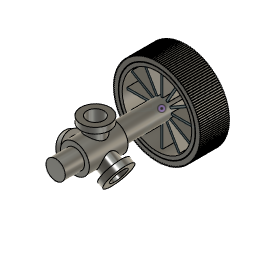
Inner Rotor Generator + Hub (Autodesk Fusion 360 design; units mm, degrees)
Autodesk Fusion 360 part; units mm, degrees
(part 1 of 2)
sketch "Sketch1" plane through (0, 0, 0) normal (0, 1, 0) x (1, 0, 0) in component "Inner Rotor Generator"
  circle A0 centre (0, 0) radius 4500
  circle A1 centre (0, 0) radius 4000
  circle A2 centre (0, 0) radius 1000
  circle A3 centre (0, 0) radius 3950
  circle A4 centre (0, 0) radius 3600
  line L0 (-100, -900) -> (100, -900)
  line L1 (100, -900) -> (100, -3700)
  line L2 (100, -3700) -> (-100, -3700)
  line L3 (-100, -3700) -> (-100, -900)
  line L4 (20.1805, -4430.0009) -> (-19.8217, -4429.9984)
  line L5 (-19.8217, -4429.9984) -> (-19.8172, -4499.9564)
  line L6 (20.176, -4499.9548) -> (20.1805, -4430.0009)
  line L7 (-19.8172, -4499.9564) -> (20.176, -4499.9548)
  line L8 (165.7048, -4426.9426) -> (168.6388, -4496.839)
  line L9 (168.6388, -4496.839) -> (208.5969, -4495.1627)
  line L10 (208.5969, -4495.1627) -> (205.6719, -4425.27)
  line L11 (205.6719, -4425.27) -> (165.7048, -4426.9426)
  line L12 (350.9405, -4416.1204) -> (356.7989, -4485.8326)
  line L13 (356.7989, -4485.8326) -> (396.6518, -4482.4845)
  line L14 (396.6518, -4482.4845) -> (390.8026, -4412.7756)
  line L15 (390.8026, -4412.7756) -> (350.9405, -4416.1204)
  line L16 (535.5606, -4397.5508) -> (544.3331, -4466.9566)
  line L17 (544.3331, -4466.9566) -> (584.0108, -4461.9426)
  line L18 (584.0108, -4461.9426) -> (575.2477, -4392.5398)
  line L19 (575.2477, -4392.5398) -> (535.5606, -4397.5508)
  line L20 (719.2411, -4371.2665) -> (730.9124, -4440.244)
  line L21 (730.9124, -4440.244) -> (770.3453, -4433.5728)
  line L22 (770.3453, -4433.5728) -> (758.6836, -4364.5979)
  line L23 (758.6836, -4364.5979) -> (719.2411, -4371.2665)
  line L24 (901.6599, -4337.3135) -> (916.2094, -4405.7417)
  line L25 (916.2094, -4405.7417) -> (955.3283, -4397.4251)
  line L26 (955.3283, -4397.4251) -> (940.7885, -4328.999)
  line L27 (940.7885, -4328.999) -> (901.6599, -4337.3135)
  line L28 (1082.4968, -4295.7513) -> (1099.899, -4363.5103)
  line L29 (1099.899, -4363.5103) -> (1138.6354, -4353.5628)
  line L30 (1138.6354, -4353.5628) -> (1121.2429, -4285.8056)
  line L31 (1121.2429, -4285.8056) -> (1082.4968, -4295.7513)
  line L32 (1261.4347, -4246.6529) -> (1281.6591, -4313.6238)
  line L33 (1281.6591, -4313.6238) -> (1319.9449, -4302.0629)
  line L34 (1319.9449, -4302.0629) -> (1299.7303, -4235.0935)
  line L35 (1299.7303, -4235.0935) -> (1261.4347, -4246.6529)
  line L36 (1438.1596, -4190.1045) -> (1461.1707, -4256.1697)
  line L37 (1461.1707, -4256.1697) -> (1498.9388, -4243.0157)
  line L38 (1498.9388, -4243.0157) -> (1475.9375, -4176.9515)
  line L39 (1475.9375, -4176.9515) -> (1438.1596, -4190.1045)
  line L40 (1612.3614, -4126.2052) -> (1638.1189, -4191.2488)
  line L41 (1638.1189, -4191.2488) -> (1675.303, -4176.5248)
  line L42 (1675.303, -4176.5248) -> (1649.5554, -4111.4818)
  line L43 (1649.5554, -4111.4818) -> (1612.3614, -4126.2052)
  line L44 (1783.7346, -4055.0671) -> (1812.1932, -4118.9751)
  line L45 (1812.1932, -4118.9751) -> (1848.7282, -4102.7069)
  line L46 (1848.7282, -4102.7069) -> (1820.2795, -4038.7991)
  line L47 (1820.2795, -4038.7991) -> (1783.7346, -4055.0671)
  line L48 (1951.9786, -3976.8151) -> (1983.0884, -4039.4753)
  line L49 (1983.0884, -4039.4753) -> (2018.9101, -4021.6914)
  line L50 (2018.9101, -4021.6914) -> (1987.8101, -3959.031)
  line L51 (1987.8101, -3959.031) -> (1951.9786, -3976.8151)
  line L52 (2116.7981, -3891.5864) -> (2150.5046, -3952.8888)
  line L53 (2150.5046, -3952.8888) -> (2185.5501, -3933.6205)
  line L54 (2185.5501, -3933.6205) -> (2151.8535, -3872.3174)
  line L55 (2151.8535, -3872.3174) -> (2116.7981, -3891.5864)
  line L56 (2277.904, -3799.5305) -> (2314.148, -3859.3677)
  line L57 (2314.148, -3859.3677) -> (2348.356, -3838.6488)
  line L58 (2348.356, -3838.6488) -> (2312.1218, -3778.8104)
  line L59 (2312.1218, -3778.8104) -> (2277.904, -3799.5305)
  line L60 (2435.0137, -3700.8089) -> (2473.7317, -3759.0759)
  line L61 (2473.7317, -3759.0759) -> (2507.042, -3736.9427)
  line L62 (2507.042, -3736.9427) -> (2468.3338, -3678.6742)
  line L63 (2468.3338, -3678.6742) -> (2435.0137, -3700.8089)
  line L64 (2587.8516, -3595.5949) -> (2628.9755, -3652.1894)
  line L65 (2628.9755, -3652.1894) -> (2661.3298, -3628.6807)
  line L66 (2661.3298, -3628.6807) -> (2620.2156, -3572.0843)
  line L67 (2620.2156, -3572.0843) -> (2587.8516, -3595.5949)
  line L68 (2736.1495, -3484.073) -> (2779.6073, -3538.8958)
  line L69 (2779.6073, -3538.8958) -> (2810.9487, -3514.0528)
  line L70 (2810.9487, -3514.0528) -> (2767.5005, -3459.2277)
  line L71 (2767.5005, -3459.2277) -> (2736.1495, -3484.073)
  line L72 (2879.6473, -3366.4388) -> (2925.3627, -3419.3937)
  line L73 (2925.3627, -3419.3937) -> (2955.6363, -3393.2601)
  line L74 (2955.6363, -3393.2601) -> (2909.9304, -3340.3025)
  line L75 (2909.9304, -3340.3025) -> (2879.6473, -3366.4388)
  line L76 (3018.0932, -3242.8987) -> (3065.986, -3293.8928)
  line L77 (3065.986, -3293.8928) -> (3095.1387, -3266.5144)
  line L78 (3095.1387, -3266.5144) -> (3047.2552, -3215.5172)
  line L79 (3047.2552, -3215.5172) -> (3018.0932, -3242.8987)
  line L80 (3151.2443, -3113.6695) -> (3201.2305, -3162.6133)
  line L81 (3201.2305, -3162.6133) -> (3229.2112, -3134.0382)
  line L82 (3229.2112, -3134.0382) -> (3179.2342, -3085.0909)
  line L83 (3179.2342, -3085.0909) -> (3151.2443, -3113.6695)
  line L84 (3278.8671, -2978.9779) -> (3330.859, -3025.7856)
  line L85 (3330.859, -3025.7856) -> (3357.6185, -2996.0637)
  line L86 (3357.6185, -2996.0637) -> (3305.6356, -2949.2522)
  line L87 (3305.6356, -2949.2522) -> (3278.8671, -2978.9779)
  line L88 (3400.7376, -2839.0601) -> (3454.644, -2883.6496)
  line L89 (3454.644, -2883.6496) -> (3480.1354, -2852.8332)
  line L90 (3480.1354, -2852.8332) -> (3426.2379, -2808.2395)
  line L91 (3426.2379, -2808.2395) -> (3400.7376, -2839.0601)
  line L92 (3516.6421, -2694.1617) -> (3572.3684, -2736.4546)
  line L93 (3572.3684, -2736.4546) -> (3596.547, -2704.5979)
  line L94 (3596.547, -2704.5979) -> (3540.8294, -2662.3003)
  line L95 (3540.8294, -2662.3003) -> (3516.6421, -2694.1617)
  line L96 (3626.3772, -2544.5368) -> (3683.8257, -2584.459)
  line L97 (3683.8257, -2584.459) -> (3706.649, -2551.6177)
  line L98 (3706.649, -2551.6177) -> (3649.209, -2511.6905)
  line L99 (3649.209, -2511.6905) -> (3626.3772, -2544.5368)
  line L100 (3729.7503, -2390.4479) -> (3788.8202, -2427.9294)
  line L101 (3788.8202, -2427.9294) -> (3810.2483, -2394.1612)
  line L102 (3810.2483, -2394.1612) -> (3751.1867, -2356.6743)
  line L103 (3751.1867, -2356.6743) -> (3729.7503, -2390.4479)
  line L104 (3826.5803, -2232.1653) -> (3887.1679, -2267.1404)
  line L105 (3887.1679, -2267.1404) -> (3907.1632, -2232.5044)
  line L106 (3907.1632, -2232.5044) -> (3846.5836, -2197.5237)
  line L107 (3846.5836, -2197.5237) -> (3826.5803, -2232.1653)
  line L108 (3916.6971, -2069.9668) -> (3978.6962, -2102.374)
  line L109 (3978.6962, -2102.374) -> (3997.2235, -2066.9311)
  line L110 (3997.2235, -2066.9311) -> (3935.2322, -2034.5179)
  line L111 (3935.2322, -2034.5179) -> (3916.6971, -2069.9668)
  line L112 (3999.9427, -1904.1368) -> (4063.2445, -1933.9194)
  line L113 (4063.2445, -1933.9194) -> (4080.2713, -1897.7317)
  line L114 (4080.2713, -1897.7317) -> (4016.9771, -1867.9428)
  line L115 (4016.9771, -1867.9428) -> (3999.9427, -1904.1368)
  line L116 (4076.1711, -1734.9663) -> (4140.6645, -1762.072)
  line L117 (4140.6645, -1762.072) -> (4156.161, -1725.2031)
  line L118 (4156.161, -1725.2031) -> (4091.6749, -1698.0908)
  line L119 (4091.6749, -1698.0908) -> (4076.1711, -1734.9663)
  line L120 (4145.2484, -1562.7521) -> (4210.8203, -1587.1333)
  line L121 (4210.8203, -1587.1333) -> (4224.7594, -1549.6478)
  line L122 (4224.7594, -1549.6478) -> (4159.1944, -1525.2597)
  line L123 (4159.1944, -1525.2597) -> (4145.2484, -1562.7521)
  line L124 (4207.0536, -1387.7964) -> (4273.589, -1409.4103)
  line L125 (4273.589, -1409.4103) -> (4285.946, -1371.3739)
  line L126 (4285.946, -1371.3739) -> (4219.4174, -1349.7528)
  line L127 (4219.4174, -1349.7528) -> (4207.0536, -1387.7964)
  line L128 (4261.4782, -1210.4059) -> (4328.8603, -1229.2146)
  line L129 (4328.8603, -1229.2146) -> (4339.6137, -1190.6942)
  line L130 (4339.6137, -1190.6942) -> (4272.238, -1171.878)
  line L131 (4272.238, -1171.878) -> (4261.4782, -1210.4059)
  line L132 (4308.4267, -1030.892) -> (4376.5373, -1046.8626)
  line L133 (4376.5373, -1046.8626) -> (4385.6682, -1007.9256)
  line L134 (4385.6682, -1007.9256) -> (4317.5637, -991.9473)
  line L135 (4317.5637, -991.9473) -> (4308.4267, -1030.892)
  line L136 (4347.8167, -849.5695) -> (4416.5364, -862.6739)
  line L137 (4416.5364, -862.6739) -> (4424.0288, -823.3888)
  line L138 (4424.0288, -823.3888) -> (4355.3149, -810.2764)
  line L139 (4355.3149, -810.2764) -> (4347.8167, -849.5695)
  line L140 (4379.5792, -666.7567) -> (4448.7874, -676.9719)
  line L141 (4448.7874, -676.9719) -> (4454.6281, -637.4074)
  line L142 (4454.6281, -637.4074) -> (4385.4254, -627.184)
  line L143 (4385.4254, -627.184) -> (4379.5792, -666.7567)
  line L144 (4403.6585, -482.7741) -> (4473.2337, -490.0822)
  line L145 (4473.2337, -490.0822) -> (4477.4125, -450.3078)
  line L146 (4477.4125, -450.3078) -> (4407.8423, -442.9913)
  line L147 (4407.8423, -442.9913) -> (4403.6585, -482.7741)
  line L148 (4420.0122, -297.9445) -> (4489.8324, -302.3327)
  line L149 (4489.8324, -302.3327) -> (4492.342, -262.4183)
  line L150 (4492.342, -262.4183) -> (4422.5265, -258.0214)
  line L151 (4422.5265, -258.0214) -> (4420.0122, -297.9445)
  line L152 (4428.6117, -112.5923) -> (4498.5544, -114.0528)
  line L153 (4498.5544, -114.0528) -> (4499.3904, -74.0683)
  line L154 (4499.3904, -74.0683) -> (4429.452, -72.5989)
  line L155 (4429.452, -72.5989) -> (4428.6117, -112.5923)
  line L156 (4429.4419, 72.9575) -> (4499.3845, 74.4271)
  line L157 (4499.3845, 74.4271) -> (4498.5453, 114.4116)
  line L158 (4498.5453, 114.4116) -> (4428.6067, 112.951)
  line L159 (4428.6067, 112.951) -> (4429.4419, 72.9575)
  line L160 (4422.5014, 258.3793) -> (4492.3211, 262.7765)
  line L161 (4492.3211, 262.7765) -> (4489.8083, 302.6907)
  line L162 (4489.8083, 302.6907) -> (4419.9922, 298.3027)
  line L163 (4419.9922, 298.3027) -> (4422.5014, 258.3793)
  line L164 (4407.8023, 443.3478) -> (4477.3766, 450.6649)
  line L165 (4477.3766, 450.6649) -> (4473.1946, 490.4389)
  line L166 (4473.1946, 490.4389) -> (4403.6235, 483.1311)
  line L167 (4403.6235, 483.1311) -> (4407.8023, 443.3478)
  line L168 (4385.3705, 627.5385) -> (4454.5773, 637.7626)
  line L169 (4454.5773, 637.7626) -> (4448.7334, 677.3266)
  line L170 (4448.7334, 677.3266) -> (4379.5293, 667.1119)
  line L171 (4379.5293, 667.1119) -> (4385.3705, 627.5385)
  line L172 (4355.2452, 810.6283) -> (4423.9631, 823.7416)
  line L173 (4423.9631, 823.7416) -> (4416.4676, 863.0261)
  line L174 (4416.4676, 863.0261) -> (4347.752, 849.9224)
  line L175 (4347.752, 849.9224) -> (4355.2452, 810.6283)
  line L176 (4317.4793, 992.296) -> (4385.5879, 1008.2753)
  line L177 (4385.5879, 1008.2753) -> (4376.4538, 1047.2115)
  line L178 (4376.4538, 1047.2115) -> (4308.3472, 1031.2418)
  line L179 (4308.3472, 1031.2418) -> (4317.4793, 992.296)
  line L180 (4272.1391, 1172.2228) -> (4339.5188, 1191.0403)
  line L181 (4339.5188, 1191.0403) -> (4328.7623, 1229.5598)
  line L182 (4328.7623, 1229.5598) -> (4261.3841, 1210.7521)
  line L183 (4261.3841, 1210.7521) -> (4272.1391, 1172.2228)
  line L184 (4219.3041, 1350.0932) -> (4285.8367, 1371.7157)
  line L185 (4285.8367, 1371.7157) -> (4273.4766, 1409.751)
  line L186 (4273.4766, 1409.751) -> (4206.9451, 1388.1383)
  line L187 (4206.9451, 1388.1383) -> (4219.3041, 1350.0932)
  line L188 (4159.067, 1525.5951) -> (4224.6358, 1549.9847)
  line L189 (4224.6358, 1549.9847) -> (4210.6938, 1587.4691)
  line L190 (4210.6938, 1587.4691) -> (4145.1257, 1563.0893)
  line L191 (4145.1257, 1563.0893) -> (4159.067, 1525.5951)
  line L192 (4091.5335, 1698.4205) -> (4156.0234, 1725.5345)
  line L193 (4156.0234, 1725.5345) -> (4140.524, 1762.4022)
  line L194 (4140.524, 1762.4022) -> (4076.0344, 1735.298)
  line L195 (4076.0344, 1735.298) -> (4091.5335, 1698.4205)
  line L196 (4016.8221, 1868.2664) -> (4080.12, 1898.0571)
  line L197 (4080.12, 1898.0571) -> (4063.0903, 1934.2434)
  line L198 (4063.0903, 1934.2434) -> (3999.7923, 1904.4625)
  line L199 (3999.7923, 1904.4625) -> (4016.8221, 1868.2664)
  line L200 (3935.0638, 2034.8346) -> (3997.0587, 2067.2499)
  line L201 (3997.0587, 2067.2499) -> (3978.5285, 2102.6913)
  line L202 (3978.5285, 2102.6913) -> (3916.5331, 2070.2859)
  line L203 (3916.5331, 2070.2859) -> (3935.0638, 2034.8346)
  line L204 (3846.402, 2197.8331) -> (3906.9851, 2232.816)
  line L205 (3906.9851, 2232.816) -> (3886.9871, 2267.4503)
  line L206 (3886.9871, 2267.4503) -> (3826.4031, 2232.4773)
  line L207 (3826.4031, 2232.4773) -> (3846.402, 2197.8331)
  line L208 (3750.9924, 2356.9758) -> (3810.0574, 2394.465)
  line L209 (3810.0574, 2394.465) -> (3788.6266, 2428.2315)
  line L210 (3788.6266, 2428.2315) -> (3729.5603, 2390.7521)
  line L211 (3729.5603, 2390.7521) -> (3750.9924, 2356.9758)
  line L212 (3649.0022, 2511.9836) -> (3706.4456, 2551.9133)
  line L213 (3706.4456, 2551.9133) -> (3683.6196, 2584.7528)
  line L214 (3683.6196, 2584.7528) -> (3626.1745, 2544.8328)
  line L215 (3626.1745, 2544.8328) -> (3649.0022, 2511.9836)
  line L216 (3540.6104, 2662.5845) -> (3596.3313, 2704.8846)
  line L217 (3596.3313, 2704.8846) -> (3572.1502, 2736.7395)
  line L218 (3572.1502, 2736.7395) -> (3516.4272, 2694.449)
  line L219 (3516.4272, 2694.449) -> (3540.6104, 2662.5845)
  line L220 (3426.0073, 2808.5144) -> (3479.9079, 2853.1107)
  line L221 (3479.9079, 2853.1107) -> (3454.4141, 2883.925)
  line L222 (3454.4141, 2883.925) -> (3400.5109, 2839.3382)
  line L223 (3400.5109, 2839.3382) -> (3426.0073, 2808.5144)
  line L224 (3305.3937, 2949.5171) -> (3357.3796, 2996.3315)
  line L225 (3357.3796, 2996.3315) -> (3330.6177, 3026.0512)
  line L226 (3330.6177, 3026.0512) -> (3278.6289, 2979.2462)
  line L227 (3278.6289, 2979.2462) -> (3305.3937, 2949.5171)
  line L228 (3178.9813, 3085.3454) -> (3228.9612, 3134.2957)
  line L229 (3228.9612, 3134.2957) -> (3200.9783, 3162.8686)
  line L230 (3200.9783, 3162.8686) -> (3150.9951, 3113.9276)
  line L231 (3150.9951, 3113.9276) -> (3178.9813, 3085.3454)
  line L232 (3046.992, 3215.7609) -> (3094.8782, 3266.7612)
  line L233 (3094.8782, 3266.7612) -> (3065.7233, 3294.1373)
  line L234 (3065.7233, 3294.1373) -> (3017.8334, 3243.1462)
  line L235 (3017.8334, 3243.1462) -> (3046.992, 3215.7609)
  line L236 (2909.6572, 3340.535) -> (2955.3657, 3393.4958)
  line L237 (2955.3657, 3393.4958) -> (2925.09, 3419.6269)
  line L238 (2925.09, 3419.6269) -> (2879.3774, 3366.6751)
  line L239 (2879.3774, 3366.6751) -> (2909.6572, 3340.535)
  line L240 (2767.2178, 3459.4485) -> (2810.6685, 3514.277)
  line L241 (2810.6685, 3514.277) -> (2779.3251, 3539.1174)
  line L242 (2779.3251, 3539.1174) -> (2735.8699, 3484.2978)
  line L243 (2735.8699, 3484.2978) -> (2767.2178, 3459.4485)
  line L244 (2619.9238, 3572.2931) -> (2661.0404, 3628.8929)
  line L245 (2661.0404, 3628.8929) -> (2628.6843, 3652.3991)
  line L246 (2628.6843, 3652.3991) -> (2587.5629, 3595.8078)
  line L247 (2587.5629, 3595.8078) -> (2619.9238, 3572.2931)
  line L248 (2468.0336, 3678.8706) -> (2506.744, 3737.1426)
  line L249 (2506.744, 3737.1426) -> (2473.4319, 3759.2732)
  line L250 (2473.4319, 3759.2732) -> (2434.7163, 3701.0096)
  line L251 (2434.7163, 3701.0096) -> (2468.0336, 3678.8706)
  line L252 (2311.8136, 3778.9941) -> (2348.0499, 3838.836)
  line L253 (2348.0499, 3838.836) -> (2313.8403, 3859.5522)
  line L254 (2313.8403, 3859.5522) -> (2277.5985, 3799.7185)
  line L255 (2277.5985, 3799.7185) -> (2311.8136, 3778.9941)
  line L256 (2151.5379, 3872.488) -> (2185.2365, 3933.7948)
  line L257 (2185.2365, 3933.7948) -> (2150.1894, 3953.0603)
  line L258 (2150.1894, 3953.0603) -> (2116.4849, 3891.7614)
  line L259 (2116.4849, 3891.7614) -> (2151.5379, 3872.488)
  line L260 (1987.4877, 3959.1882) -> (2018.5894, 4021.8524)
  line L261 (2018.5894, 4021.8524) -> (1982.7663, 4039.6334)
  line L262 (1982.7663, 4039.6334) -> (1951.6584, 3976.9769)
  line L263 (1951.6584, 3976.9769) -> (1987.4877, 3959.1882)
  line L264 (1819.9507, 4038.9427) -> (1848.4011, 4102.8543)
  line L265 (1848.4011, 4102.8543) -> (1811.8648, 4119.1196)
  line L266 (1811.8648, 4119.1196) -> (1783.4079, 4055.2154)
  line L267 (1783.4079, 4055.2154) -> (1819.9507, 4038.9427)
  line L268 (1649.2209, 4111.6115) -> (1674.97, 4176.6584)
  line L269 (1674.97, 4176.6584) -> (1637.7846, 4191.3794)
  line L270 (1637.7846, 4191.3794) -> (1612.0288, 4126.3396)
  line L271 (1612.0288, 4126.3396) -> (1649.2209, 4111.6115)
  line L272 (1475.5979, 4177.0671) -> (1498.6005, 4243.1352)
  line L273 (1498.6005, 4243.1352) -> (1460.8313, 4256.2862)
  line L274 (1460.8313, 4256.2862) -> (1437.8216, 4190.2249)
  line L275 (1437.8216, 4190.2249) -> (1475.5979, 4177.0671)
  line L276 (1299.3861, 4235.1947) -> (1319.6019, 4302.1682)
  line L277 (1319.6019, 4302.1682) -> (1281.3151, 4313.726)
  line L278 (1281.3151, 4313.726) -> (1261.092, 4246.7591)
  line L279 (1261.092, 4246.7591) -> (1299.3861, 4235.1947)
  line L280 (1120.8948, 4285.8924) -> (1138.2882, 4353.6536)
  line L281 (1138.2882, 4353.6536) -> (1099.5511, 4363.598)
  line L282 (1099.5511, 4363.598) -> (1082.15, 4295.843)
  line L283 (1082.15, 4295.843) -> (1120.8948, 4285.8924)
  line L284 (940.437, 4329.0711) -> (954.9777, 4397.5013)
  line L285 (954.9777, 4397.5013) -> (915.8581, 4405.8148)
  line L286 (915.8581, 4405.8148) -> (901.3095, 4337.3905)
  line L287 (901.3095, 4337.3905) -> (940.437, 4329.0711)
  line L288 (758.3294, 4364.6552) -> (769.9918, 4433.6343)
  line L289 (769.9918, 4433.6343) -> (730.5583, 4440.3023)
  line L290 (730.5583, 4440.3023) -> (718.8878, 4371.3288)
  line L291 (718.8878, 4371.3288) -> (758.3294, 4364.6552)
  line L292 (574.8914, 4392.5822) -> (583.655, 4461.9891)
  line L293 (583.655, 4461.9891) -> (543.9769, 4467)
  line L294 (543.9769, 4467) -> (535.205, 4397.5983)
  line L295 (535.205, 4397.5983) -> (574.8914, 4392.5822)
  line L296 (390.4449, 4412.8031) -> (396.2943, 4482.5161)
  line L297 (396.2943, 4482.5161) -> (356.4412, 4485.8611)
  line L298 (356.4412, 4485.8611) -> (350.5832, 4416.1529)
  line L299 (350.5832, 4416.1529) -> (390.4449, 4412.8031)
  line L300 (205.3134, 4425.2825) -> (208.2384, 4495.1793)
  line L301 (208.2384, 4495.1793) -> (168.2802, 4496.8524)
  line L302 (168.2802, 4496.8524) -> (165.3464, 4426.9601)
  line L303 (165.3464, 4426.9601) -> (205.3134, 4425.2825)
  line L304 (19.8217, 4429.9984) -> (19.8172, 4499.9564)
  line L305 (19.8172, 4499.9564) -> (-20.176, 4499.9548)
  line L306 (-20.176, 4499.9548) -> (-20.1805, 4430.0009)
  line L307 (-20.1805, 4430.0009) -> (19.8217, 4429.9984)
  line L308 (-165.7048, 4426.9426) -> (-168.6388, 4496.839)
  line L309 (-168.6388, 4496.839) -> (-208.5969, 4495.1627)
  line L310 (-208.5969, 4495.1627) -> (-205.6719, 4425.27)
  line L311 (-205.6719, 4425.27) -> (-165.7048, 4426.9426)
  line L312 (-350.9405, 4416.1204) -> (-356.7989, 4485.8326)
  line L313 (-356.7989, 4485.8326) -> (-396.6518, 4482.4845)
  line L314 (-396.6518, 4482.4845) -> (-390.8026, 4412.7756)
  line L315 (-390.8026, 4412.7756) -> (-350.9405, 4416.1204)
  line L316 (-535.5606, 4397.5508) -> (-544.3331, 4466.9566)
  line L317 (-544.3331, 4466.9566) -> (-584.0108, 4461.9426)
  line L318 (-584.0108, 4461.9426) -> (-575.2477, 4392.5398)
  line L319 (-575.2477, 4392.5398) -> (-535.5606, 4397.5508)
  line L320 (-719.2411, 4371.2665) -> (-730.9124, 4440.244)
  line L321 (-730.9124, 4440.244) -> (-770.3453, 4433.5728)
  line L322 (-770.3453, 4433.5728) -> (-758.6836, 4364.5979)
  line L323 (-758.6836, 4364.5979) -> (-719.2411, 4371.2665)
  line L324 (-901.6599, 4337.3135) -> (-916.2094, 4405.7417)
  line L325 (-916.2094, 4405.7417) -> (-955.3283, 4397.4251)
  line L326 (-955.3283, 4397.4251) -> (-940.7885, 4328.999)
  line L327 (-940.7885, 4328.999) -> (-901.6599, 4337.3135)
  line L328 (-1082.4968, 4295.7513) -> (-1099.899, 4363.5103)
  line L329 (-1099.899, 4363.5103) -> (-1138.6354, 4353.5628)
  line L330 (-1138.6354, 4353.5628) -> (-1121.2429, 4285.8056)
  line L331 (-1121.2429, 4285.8056) -> (-1082.4968, 4295.7513)
  line L332 (-1261.4347, 4246.6529) -> (-1281.6591, 4313.6238)
  line L333 (-1281.6591, 4313.6238) -> (-1319.9449, 4302.0629)
  line L334 (-1319.9449, 4302.0629) -> (-1299.7303, 4235.0935)
  line L335 (-1299.7303, 4235.0935) -> (-1261.4347, 4246.6529)
  line L336 (-1438.1596, 4190.1045) -> (-1461.1707, 4256.1697)
  line L337 (-1461.1707, 4256.1697) -> (-1498.9388, 4243.0157)
  line L338 (-1498.9388, 4243.0157) -> (-1475.9375, 4176.9515)
  line L339 (-1475.9375, 4176.9515) -> (-1438.1596, 4190.1045)
  line L340 (-1612.3614, 4126.2052) -> (-1638.1189, 4191.2488)
  line L341 (-1638.1189, 4191.2488) -> (-1675.303, 4176.5248)
  line L342 (-1675.303, 4176.5248) -> (-1649.5554, 4111.4818)
  line L343 (-1649.5554, 4111.4818) -> (-1612.3614, 4126.2052)
  line L344 (-1783.7346, 4055.0671) -> (-1812.1932, 4118.9751)
  line L345 (-1812.1932, 4118.9751) -> (-1848.7282, 4102.7069)
  line L346 (-1848.7282, 4102.7069) -> (-1820.2795, 4038.7991)
  line L347 (-1820.2795, 4038.7991) -> (-1783.7346, 4055.0671)
  line L348 (-1951.9786, 3976.8151) -> (-1983.0884, 4039.4753)
  line L349 (-1983.0884, 4039.4753) -> (-2018.9101, 4021.6914)
  line L350 (-2018.9101, 4021.6914) -> (-1987.8101, 3959.031)
  line L351 (-1987.8101, 3959.031) -> (-1951.9786, 3976.8151)
  line L352 (-2116.7981, 3891.5864) -> (-2150.5046, 3952.8888)
  line L353 (-2150.5046, 3952.8888) -> (-2185.5501, 3933.6205)
  line L354 (-2185.5501, 3933.6205) -> (-2151.8535, 3872.3174)
  line L355 (-2151.8535, 3872.3174) -> (-2116.7981, 3891.5864)
  line L356 (-2277.904, 3799.5305) -> (-2314.148, 3859.3677)
  line L357 (-2314.148, 3859.3677) -> (-2348.356, 3838.6488)
  line L358 (-2348.356, 3838.6488) -> (-2312.1218, 3778.8104)
  line L359 (-2312.1218, 3778.8104) -> (-2277.904, 3799.5305)
  line L360 (-2435.0137, 3700.8089) -> (-2473.7317, 3759.0759)
  line L361 (-2473.7317, 3759.0759) -> (-2507.042, 3736.9427)
  line L362 (-2507.042, 3736.9427) -> (-2468.3338, 3678.6742)
  line L363 (-2468.3338, 3678.6742) -> (-2435.0137, 3700.8089)
  line L364 (-2587.8516, 3595.5949) -> (-2628.9755, 3652.1894)
  line L365 (-2628.9755, 3652.1894) -> (-2661.3298, 3628.6807)
  line L366 (-2661.3298, 3628.6807) -> (-2620.2156, 3572.0843)
  line L367 (-2620.2156, 3572.0843) -> (-2587.8516, 3595.5949)
  line L368 (-2736.1495, 3484.073) -> (-2779.6073, 3538.8958)
  line L369 (-2779.6073, 3538.8958) -> (-2810.9487, 3514.0528)
  line L370 (-2810.9487, 3514.0528) -> (-2767.5005, 3459.2277)
  line L371 (-2767.5005, 3459.2277) -> (-2736.1495, 3484.073)
  line L372 (-2879.6473, 3366.4388) -> (-2925.3627, 3419.3937)
  line L373 (-2925.3627, 3419.3937) -> (-2955.6363, 3393.2601)
  line L374 (-2955.6363, 3393.2601) -> (-2909.9304, 3340.3025)
  line L375 (-2909.9304, 3340.3025) -> (-2879.6473, 3366.4388)
  line L376 (-3018.0932, 3242.8987) -> (-3065.986, 3293.8928)
  line L377 (-3065.986, 3293.8928) -> (-3095.1387, 3266.5144)
  line L378 (-3095.1387, 3266.5144) -> (-3047.2552, 3215.5172)
  line L379 (-3047.2552, 3215.5172) -> (-3018.0932, 3242.8987)
  line L380 (-3151.2443, 3113.6695) -> (-3201.2305, 3162.6133)
  line L381 (-3201.2305, 3162.6133) -> (-3229.2112, 3134.0382)
  line L382 (-3229.2112, 3134.0382) -> (-3179.2342, 3085.0909)
  line L383 (-3179.2342, 3085.0909) -> (-3151.2443, 3113.6695)
  line L384 (-3278.8671, 2978.9779) -> (-3330.859, 3025.7856)
  line L385 (-3330.859, 3025.7856) -> (-3357.6185, 2996.0637)
  line L386 (-3357.6185, 2996.0637) -> (-3305.6356, 2949.2522)
  line L387 (-3305.6356, 2949.2522) -> (-3278.8671, 2978.9779)
  line L388 (-3400.7376, 2839.0601) -> (-3454.644, 2883.6496)
  line L389 (-3454.644, 2883.6496) -> (-3480.1354, 2852.8332)
  line L390 (-3480.1354, 2852.8332) -> (-3426.2379, 2808.2395)
  line L391 (-3426.2379, 2808.2395) -> (-3400.7376, 2839.0601)
  line L392 (-3516.6421, 2694.1617) -> (-3572.3684, 2736.4546)
  line L393 (-3572.3684, 2736.4546) -> (-3596.547, 2704.5979)
  line L394 (-3596.547, 2704.5979) -> (-3540.8294, 2662.3003)
  line L395 (-3540.8294, 2662.3003) -> (-3516.6421, 2694.1617)
  line L396 (-3626.3772, 2544.5368) -> (-3683.8257, 2584.459)
  line L397 (-3683.8257, 2584.459) -> (-3706.649, 2551.6177)
  line L398 (-3706.649, 2551.6177) -> (-3649.209, 2511.6905)
  line L399 (-3649.209, 2511.6905) -> (-3626.3772, 2544.5368)
  line L400 (-3729.7503, 2390.4479) -> (-3788.8202, 2427.9294)
  line L401 (-3788.8202, 2427.9294) -> (-3810.2483, 2394.1612)
  line L402 (-3810.2483, 2394.1612) -> (-3751.1867, 2356.6743)
  line L403 (-3751.1867, 2356.6743) -> (-3729.7503, 2390.4479)
  line L404 (-3826.5803, 2232.1653) -> (-3887.1679, 2267.1404)
  line L405 (-3887.1679, 2267.1404) -> (-3907.1632, 2232.5044)
  line L406 (-3907.1632, 2232.5044) -> (-3846.5836, 2197.5237)
  line L407 (-3846.5836, 2197.5237) -> (-3826.5803, 2232.1653)
  line L408 (-3916.6971, 2069.9668) -> (-3978.6962, 2102.374)
  line L409 (-3978.6962, 2102.374) -> (-3997.2235, 2066.9311)
  line L410 (-3997.2235, 2066.9311) -> (-3935.2322, 2034.5179)
  line L411 (-3935.2322, 2034.5179) -> (-3916.6971, 2069.9668)
  line L412 (-3999.9427, 1904.1368) -> (-4063.2445, 1933.9194)
  line L413 (-4063.2445, 1933.9194) -> (-4080.2713, 1897.7317)
  line L414 (-4080.2713, 1897.7317) -> (-4016.9771, 1867.9428)
  line L415 (-4016.9771, 1867.9428) -> (-3999.9427, 1904.1368)
  line L416 (-4076.1711, 1734.9663) -> (-4140.6645, 1762.072)
  line L417 (-4140.6645, 1762.072) -> (-4156.161, 1725.2031)
  line L418 (-4156.161, 1725.2031) -> (-4091.6749, 1698.0908)
  line L419 (-4091.6749, 1698.0908) -> (-4076.1711, 1734.9663)
  line L420 (-4145.2484, 1562.7521) -> (-4210.8203, 1587.1333)
  line L421 (-4210.8203, 1587.1333) -> (-4224.7594, 1549.6478)
  line L422 (-4224.7594, 1549.6478) -> (-4159.1944, 1525.2597)
  line L423 (-4159.1944, 1525.2597) -> (-4145.2484, 1562.7521)
  line L424 (-4207.0536, 1387.7964) -> (-4273.589, 1409.4103)
  line L425 (-4273.589, 1409.4103) -> (-4285.946, 1371.3739)
  line L426 (-4285.946, 1371.3739) -> (-4219.4174, 1349.7528)
  line L427 (-4219.4174, 1349.7528) -> (-4207.0536, 1387.7964)
  line L428 (-4261.4782, 1210.4059) -> (-4328.8603, 1229.2146)
  line L429 (-4328.8603, 1229.2146) -> (-4339.6137, 1190.6942)
  line L430 (-4339.6137, 1190.6942) -> (-4272.238, 1171.878)
  line L431 (-4272.238, 1171.878) -> (-4261.4782, 1210.4059)
  line L432 (-4308.4267, 1030.892) -> (-4376.5373, 1046.8626)
  line L433 (-4376.5373, 1046.8626) -> (-4385.6682, 1007.9256)
  line L434 (-4385.6682, 1007.9256) -> (-4317.5637, 991.9473)
  line L435 (-4317.5637, 991.9473) -> (-4308.4267, 1030.892)
  line L436 (-4347.8167, 849.5695) -> (-4416.5364, 862.6739)
  line L437 (-4416.5364, 862.6739) -> (-4424.0288, 823.3888)
  line L438 (-4424.0288, 823.3888) -> (-4355.3149, 810.2764)
  line L439 (-4355.3149, 810.2764) -> (-4347.8167, 849.5695)
  line L440 (-4379.5792, 666.7567) -> (-4448.7874, 676.9719)
  line L441 (-4448.7874, 676.9719) -> (-4454.6281, 637.4074)
  line L442 (-4454.6281, 637.4074) -> (-4385.4254, 627.184)
  line L443 (-4385.4254, 627.184) -> (-4379.5792, 666.7567)
  line L444 (-4403.6585, 482.7741) -> (-4473.2337, 490.0822)
  line L445 (-4473.2337, 490.0822) -> (-4477.4125, 450.3078)
  line L446 (-4477.4125, 450.3078) -> (-4407.8423, 442.9913)
  line L447 (-4407.8423, 442.9913) -> (-4403.6585, 482.7741)
  line L448 (-4420.0122, 297.9445) -> (-4489.8324, 302.3327)
  line L449 (-4489.8324, 302.3327) -> (-4492.342, 262.4183)
  line L450 (-4492.342, 262.4183) -> (-4422.5265, 258.0214)
  line L451 (-4422.5265, 258.0214) -> (-4420.0122, 297.9445)
  line L452 (-4428.6117, 112.5923) -> (-4498.5544, 114.0528)
  line L453 (-4498.5544, 114.0528) -> (-4499.3904, 74.0683)
  line L454 (-4499.3904, 74.0683) -> (-4429.452, 72.5989)
  line L455 (-4429.452, 72.5989) -> (-4428.6117, 112.5923)
  line L456 (-4429.4419, -72.9575) -> (-4499.3845, -74.4271)
  line L457 (-4499.3845, -74.4271) -> (-4498.5453, -114.4116)
  line L458 (-4498.5453, -114.4116) -> (-4428.6067, -112.951)
  line L459 (-4428.6067, -112.951) -> (-4429.4419, -72.9575)
  line L460 (-4422.5014, -258.3793) -> (-4492.3211, -262.7765)
  line L461 (-4492.3211, -262.7765) -> (-4489.8083, -302.6907)
  line L462 (-4489.8083, -302.6907) -> (-4419.9922, -298.3027)
  line L463 (-4419.9922, -298.3027) -> (-4422.5014, -258.3793)
  line L464 (-4407.8023, -443.3478) -> (-4477.3766, -450.6649)
  line L465 (-4477.3766, -450.6649) -> (-4473.1946, -490.4389)
  line L466 (-4473.1946, -490.4389) -> (-4403.6235, -483.1311)
  line L467 (-4403.6235, -483.1311) -> (-4407.8023, -443.3478)
  line L468 (-4385.3705, -627.5385) -> (-4454.5773, -637.7626)
  line L469 (-4454.5773, -637.7626) -> (-4448.7334, -677.3266)
  line L470 (-4448.7334, -677.3266) -> (-4379.5293, -667.1119)
  line L471 (-4379.5293, -667.1119) -> (-4385.3705, -627.5385)
  line L472 (-4355.2452, -810.6283) -> (-4423.9631, -823.7416)
  line L473 (-4423.9631, -823.7416) -> (-4416.4676, -863.0261)
  line L474 (-4416.4676, -863.0261) -> (-4347.752, -849.9224)
  line L475 (-4347.752, -849.9224) -> (-4355.2452, -810.6283)
  line L476 (-4317.4793, -992.296) -> (-4385.5879, -1008.2753)
  line L477 (-4385.5879, -1008.2753) -> (-4376.4538, -1047.2115)
  line L478 (-4376.4538, -1047.2115) -> (-4308.3472, -1031.2418)
  line L479 (-4308.3472, -1031.2418) -> (-4317.4793, -992.296)
  line L480 (-4272.1391, -1172.2228) -> (-4339.5188, -1191.0403)
  line L481 (-4339.5188, -1191.0403) -> (-4328.7623, -1229.5598)
  line L482 (-4328.7623, -1229.5598) -> (-4261.3841, -1210.7521)
  line L483 (-4261.3841, -1210.7521) -> (-4272.1391, -1172.2228)
  line L484 (-4219.3041, -1350.0932) -> (-4285.8367, -1371.7157)
  line L485 (-4285.8367, -1371.7157) -> (-4273.4766, -1409.751)
  line L486 (-4273.4766, -1409.751) -> (-4206.9451, -1388.1383)
  line L487 (-4206.9451, -1388.1383) -> (-4219.3041, -1350.0932)
  line L488 (-4159.067, -1525.5951) -> (-4224.6358, -1549.9847)
  line L489 (-4224.6358, -1549.9847) -> (-4210.6938, -1587.4691)
  line L490 (-4210.6938, -1587.4691) -> (-4145.1257, -1563.0893)
  line L491 (-4145.1257, -1563.0893) -> (-4159.067, -1525.5951)
  line L492 (-4091.5335, -1698.4205) -> (-4156.0234, -1725.5345)
  line L493 (-4156.0234, -1725.5345) -> (-4140.524, -1762.4022)
  line L494 (-4140.524, -1762.4022) -> (-4076.0344, -1735.298)
  line L495 (-4076.0344, -1735.298) -> (-4091.5335, -1698.4205)
  line L496 (-4016.8221, -1868.2664) -> (-4080.12, -1898.0571)
  line L497 (-4080.12, -1898.0571) -> (-4063.0903, -1934.2434)
  line L498 (-4063.0903, -1934.2434) -> (-3999.7923, -1904.4625)
  line L499 (-3999.7923, -1904.4625) -> (-4016.8221, -1868.2664)
  line L500 (-3935.0638, -2034.8346) -> (-3997.0587, -2067.2499)
  line L501 (-3997.0587, -2067.2499) -> (-3978.5285, -2102.6913)
  line L502 (-3978.5285, -2102.6913) -> (-3916.5331, -2070.2859)
  line L503 (-3916.5331, -2070.2859) -> (-3935.0638, -2034.8346)
  line L504 (-3846.402, -2197.8331) -> (-3906.9851, -2232.816)
  line L505 (-3906.9851, -2232.816) -> (-3886.9871, -2267.4503)
  line L506 (-3886.9871, -2267.4503) -> (-3826.4031, -2232.4773)
  line L507 (-3826.4031, -2232.4773) -> (-3846.402, -2197.8331)
  line L508 (-3750.9924, -2356.9758) -> (-3810.0574, -2394.465)
  line L509 (-3810.0574, -2394.465) -> (-3788.6266, -2428.2315)
  line L510 (-3788.6266, -2428.2315) -> (-3729.5603, -2390.7521)
  line L511 (-3729.5603, -2390.7521) -> (-3750.9924, -2356.9758)
  line L512 (-3649.0022, -2511.9836) -> (-3706.4456, -2551.9133)
  line L513 (-3706.4456, -2551.9133) -> (-3683.6196, -2584.7528)
  line L514 (-3683.6196, -2584.7528) -> (-3626.1745, -2544.8328)
  line L515 (-3626.1745, -2544.8328) -> (-3649.0022, -2511.9836)
  line L516 (-3540.6104, -2662.5845) -> (-3596.3313, -2704.8846)
  line L517 (-3596.3313, -2704.8846) -> (-3572.1502, -2736.7395)
  line L518 (-3572.1502, -2736.7395) -> (-3516.4272, -2694.449)
  line L519 (-3516.4272, -2694.449) -> (-3540.6104, -2662.5845)
  line L520 (-3426.0073, -2808.5144) -> (-3479.9079, -2853.1107)
  line L521 (-3479.9079, -2853.1107) -> (-3454.4141, -2883.925)
  line L522 (-3454.4141, -2883.925) -> (-3400.5109, -2839.3382)
  line L523 (-3400.5109, -2839.3382) -> (-3426.0073, -2808.5144)
  line L524 (-3305.3937, -2949.5171) -> (-3357.3796, -2996.3315)
  line L525 (-3357.3796, -2996.3315) -> (-3330.6177, -3026.0512)
  line L526 (-3330.6177, -3026.0512) -> (-3278.6289, -2979.2462)
  line L527 (-3278.6289, -2979.2462) -> (-3305.3937, -2949.5171)
  line L528 (-3178.9813, -3085.3454) -> (-3228.9612, -3134.2957)
  line L529 (-3228.9612, -3134.2957) -> (-3200.9783, -3162.8686)
  line L530 (-3200.9783, -3162.8686) -> (-3150.9951, -3113.9276)
  line L531 (-3150.9951, -3113.9276) -> (-3178.9813, -3085.3454)
  line L532 (-3046.992, -3215.7609) -> (-3094.8782, -3266.7612)
  line L533 (-3094.8782, -3266.7612) -> (-3065.7233, -3294.1373)
  line L534 (-3065.7233, -3294.1373) -> (-3017.8334, -3243.1462)
  line L535 (-3017.8334, -3243.1462) -> (-3046.992, -3215.7609)
  line L536 (-2909.6572, -3340.535) -> (-2955.3657, -3393.4958)
  line L537 (-2955.3657, -3393.4958) -> (-2925.09, -3419.6269)
  line L538 (-2925.09, -3419.6269) -> (-2879.3774, -3366.6751)
  line L539 (-2879.3774, -3366.6751) -> (-2909.6572, -3340.535)
  line L540 (-2767.2178, -3459.4485) -> (-2810.6685, -3514.277)
  line L541 (-2810.6685, -3514.277) -> (-2779.3251, -3539.1174)
  line L542 (-2779.3251, -3539.1174) -> (-2735.8699, -3484.2978)
  line L543 (-2735.8699, -3484.2978) -> (-2767.2178, -3459.4485)
  line L544 (-2619.9238, -3572.2931) -> (-2661.0404, -3628.8929)
  line L545 (-2661.0404, -3628.8929) -> (-2628.6843, -3652.3991)
  line L546 (-2628.6843, -3652.3991) -> (-2587.5629, -3595.8078)
  line L547 (-2587.5629, -3595.8078) -> (-2619.9238, -3572.2931)
  line L548 (-2468.0336, -3678.8706) -> (-2506.744, -3737.1426)
  line L549 (-2506.744, -3737.1426) -> (-2473.4319, -3759.2732)
  line L550 (-2473.4319, -3759.2732) -> (-2434.7163, -3701.0096)
  line L551 (-2434.7163, -3701.0096) -> (-2468.0336, -3678.8706)
  line L552 (-2311.8136, -3778.9941) -> (-2348.0499, -3838.836)
  line L553 (-2348.0499, -3838.836) -> (-2313.8403, -3859.5522)
  line L554 (-2313.8403, -3859.5522) -> (-2277.5985, -3799.7185)
  line L555 (-2277.5985, -3799.7185) -> (-2311.8136, -3778.9941)
  line L556 (-2151.5379, -3872.488) -> (-2185.2365, -3933.7948)
  line L557 (-2185.2365, -3933.7948) -> (-2150.1894, -3953.0603)
  line L558 (-2150.1894, -3953.0603) -> (-2116.4849, -3891.7614)
  line L559 (-2116.4849, -3891.7614) -> (-2151.5379, -3872.488)
  line L560 (-1987.4877, -3959.1882) -> (-2018.5894, -4021.8524)
  line L561 (-2018.5894, -4021.8524) -> (-1982.7663, -4039.6334)
  line L562 (-1982.7663, -4039.6334) -> (-1951.6584, -3976.9769)
  line L563 (-1951.6584, -3976.9769) -> (-1987.4877, -3959.1882)
  line L564 (-1819.9507, -4038.9427) -> (-1848.4011, -4102.8543)
  line L565 (-1848.4011, -4102.8543) -> (-1811.8648, -4119.1196)
  line L566 (-1811.8648, -4119.1196) -> (-1783.4079, -4055.2154)
  line L567 (-1783.4079, -4055.2154) -> (-1819.9507, -4038.9427)
  line L568 (-1649.2209, -4111.6115) -> (-1674.97, -4176.6584)
  line L569 (-1674.97, -4176.6584) -> (-1637.7846, -4191.3794)
  line L570 (-1637.7846, -4191.3794) -> (-1612.0288, -4126.3396)
  line L571 (-1612.0288, -4126.3396) -> (-1649.2209, -4111.6115)
  line L572 (-1475.5979, -4177.0671) -> (-1498.6005, -4243.1352)
  line L573 (-1498.6005, -4243.1352) -> (-1460.8313, -4256.2862)
  line L574 (-1460.8313, -4256.2862) -> (-1437.8216, -4190.2249)
  line L575 (-1437.8216, -4190.2249) -> (-1475.5979, -4177.0671)
  line L576 (-1299.3861, -4235.1947) -> (-1319.6019, -4302.1682)
  line L577 (-1319.6019, -4302.1682) -> (-1281.3151, -4313.726)
  line L578 (-1281.3151, -4313.726) -> (-1261.092, -4246.7591)
  line L579 (-1261.092, -4246.7591) -> (-1299.3861, -4235.1947)
  line L580 (-1120.8948, -4285.8924) -> (-1138.2882, -4353.6536)
  line L581 (-1138.2882, -4353.6536) -> (-1099.5511, -4363.598)
  line L582 (-1099.5511, -4363.598) -> (-1082.15, -4295.843)
  line L583 (-1082.15, -4295.843) -> (-1120.8948, -4285.8924)
  line L584 (-940.437, -4329.0711) -> (-954.9777, -4397.5013)
  line L585 (-954.9777, -4397.5013) -> (-915.8581, -4405.8148)
  line L586 (-915.8581, -4405.8148) -> (-901.3095, -4337.3905)
  line L587 (-901.3095, -4337.3905) -> (-940.437, -4329.0711)
  line L588 (-758.3294, -4364.6552) -> (-769.9918, -4433.6343)
  line L589 (-769.9918, -4433.6343) -> (-730.5583, -4440.3023)
  line L590 (-730.5583, -4440.3023) -> (-718.8878, -4371.3288)
  line L591 (-718.8878, -4371.3288) -> (-758.3294, -4364.6552)
  line L592 (-574.8914, -4392.5822) -> (-583.655, -4461.9891)
  line L593 (-583.655, -4461.9891) -> (-543.9769, -4467)
  line L594 (-543.9769, -4467) -> (-535.205, -4397.5983)
  line L595 (-535.205, -4397.5983) -> (-574.8914, -4392.5822)
  line L596 (-390.4449, -4412.8031) -> (-396.2943, -4482.5161)
  line L597 (-396.2943, -4482.5161) -> (-356.4412, -4485.8611)
  line L598 (-356.4412, -4485.8611) -> (-350.5832, -4416.1529)
  line L599 (-350.5832, -4416.1529) -> (-390.4449, -4412.8031)
  line L600 (-205.3134, -4425.2825) -> (-208.2384, -4495.1793)
  line L601 (-208.2384, -4495.1793) -> (-168.2802, -4496.8524)
  line L602 (-168.2802, -4496.8524) -> (-165.3464, -4426.9601)
  line L603 (-165.3464, -4426.9601) -> (-205.3134, -4425.2825)
  line L604 (536.6025, -729.4229) -> (1936.6025, -3154.294)
  line L605 (1936.6025, -3154.294) -> (1763.3975, -3254.294)
  line L606 (1763.3975, -3254.294) -> (363.3975, -829.4229)
  line L607 (363.3975, -829.4229) -> (536.6025, -729.4229)
  line L608 (829.4229, -363.3975) -> (3254.294, -1763.3975)
  line L609 (3254.294, -1763.3975) -> (3154.294, -1936.6025)
  line L610 (3154.294, -1936.6025) -> (729.4229, -536.6025)
  line L611 (729.4229, -536.6025) -> (829.4229, -363.3975)
  line L612 (900, 100) -> (3700, 100)
  line L613 (3700, 100) -> (3700, -100)
  line L614 (3700, -100) -> (900, -100)
  line L615 (900, -100) -> (900, 100)
  line L616 (729.4229, 536.6025) -> (3154.294, 1936.6025)
  line L617 (3154.294, 1936.6025) -> (3254.294, 1763.3975)
  line L618 (3254.294, 1763.3975) -> (829.4229, 363.3975)
  line L619 (829.4229, 363.3975) -> (729.4229, 536.6025)
  line L620 (363.3975, 829.4229) -> (1763.3975, 3254.294)
  line L621 (1763.3975, 3254.294) -> (1936.6025, 3154.294)
  line L622 (1936.6025, 3154.294) -> (536.6025, 729.4229)
  line L623 (536.6025, 729.4229) -> (363.3975, 829.4229)
  line L624 (-100, 900) -> (-100, 3700)
  line L625 (-100, 3700) -> (100, 3700)
  line L626 (100, 3700) -> (100, 900)
  line L627 (100, 900) -> (-100, 900)
  line L628 (-536.6025, 729.4229) -> (-1936.6025, 3154.294)
  line L629 (-1936.6025, 3154.294) -> (-1763.3975, 3254.294)
  line L630 (-1763.3975, 3254.294) -> (-363.3975, 829.4229)
  line L631 (-363.3975, 829.4229) -> (-536.6025, 729.4229)
  line L632 (-829.4229, 363.3975) -> (-3254.294, 1763.3975)
  line L633 (-3254.294, 1763.3975) -> (-3154.294, 1936.6025)
  line L634 (-3154.294, 1936.6025) -> (-729.4229, 536.6025)
  line L635 (-729.4229, 536.6025) -> (-829.4229, 363.3975)
  line L636 (-900, -100) -> (-3700, -100)
  line L637 (-3700, -100) -> (-3700, 100)
  line L638 (-3700, 100) -> (-900, 100)
  line L639 (-900, 100) -> (-900, -100)
  line L640 (-729.4229, -536.6025) -> (-3154.294, -1936.6025)
  line L641 (-3154.294, -1936.6025) -> (-3254.294, -1763.3975)
  line L642 (-3254.294, -1763.3975) -> (-829.4229, -363.3975)
  line L643 (-829.4229, -363.3975) -> (-729.4229, -536.6025)
  line L644 (-363.3975, -829.4229) -> (-1763.3975, -3254.294)
  line L645 (-1763.3975, -3254.294) -> (-1936.6025, -3154.294)
  line L646 (-1936.6025, -3154.294) -> (-536.6025, -729.4229)
  line L647 (-536.6025, -729.4229) -> (-363.3975, -829.4229)
  dimension "d5" = 360
  dimension "d7" = 360
  constraint coincident A0.centre A1.centre
  constraint concentric A0 A2
  constraint concentric A2 A3
  constraint concentric A0 A4
  constraint horizontal L0
  constraint perpendicular L0 L1
  constraint perpendicular L1 L2
  constraint perpendicular L2 L3
  constraint coincident A0 L5.end
  constraint coincident A0 L6.start
  constraint perpendicular L4 L6
extrude "Extrude1" add sketch "Sketch1" along normal blind 3000 contours A0 L4 L5 L6 L8 L10 L11 L12 L14 L15 L16 L18 L19 L20 L22 L23 L24 L26 L27 L28 L30 L31 L32 L34 L35 L36 L38 L39 L40 L42 L43 L44 L46 L47 L48 L50 L51 L52 L54 L55 L56 L58 L59 L60 L62 L63 L64 L66 L67 L68 L70 L71 L72 L74 L75 L76 L78 L79 L80 L82 L83 L84 L86 L87 L88 L90 L91 L92 L94 L95 L96 L98 L99 L100 L102 L103 L104 L106 L107 L108 L110 L111 L112 L114 L115 L116 L118 L119 L120 L122 L123 L124 L126 L127 L128 L130 L131 L132 L134 L135 L136 L138 L139 L140 L142 L143 L144 L146 L147 L148 L150 L151 L152 L154 L155 L156 L158 L159 L160 L162 L163 L164 L166 L167 L168 L170 L171 L172 L174 L175 L176 L178 L179 L180 L182 L183 L184 L186 L187 L188 L190 L191 L192 L194 L195 L196 L198 L199 L200 L202 L203 L204 L206 L207 L208 L210 L211 L212 L214 L215 L216 L218 L219 L220 L222 L223 L224 L226 L227 L228 L230 L231 L232 L234 L235 L236 L238 L239 L240 L242 L243 L244 L246 L247 L248 L250 L251 L252 L254 L255 L256 L258 L259 L260 L262 L263 L264 L266 L267 L268 L270 L271 L272 L274 L275 L276 L278 L279 L280 L282 L283 L284 L286 L287 L288 L290 L291 L292 L294 L295 L296 L298 L299 L300 L302 L303 L304 L306 L307 L308 L310 L311 L312 L314 L315 L316 L318 L319 L320 L322 L323 L324 L326 L327 L328 L330 L331 L332 L334 L335 L336 L338 L339 L340 L342 L343 L344 L346 L347 L348 L350 L351 L352 L354 L355 L356 L358 L359 L360 L362 L363 L364 L366 L367 L368 L370 L371 L372 L374 L375 L376 L378 L379 L380 L382 L383 L384 L386 L387 L388 L390 L391 L392 L394 L395 L396 L398 L399 L400 L402 L403 L404 L406 L407 L408 L410 L411 L412 L414 L415 L416 L418 L419 L420 L422 L423 L424 L426 L427 L428 L430 L431 L432 L434 L435 L436 L438 L439 L440 L442 L443 L444 L446 L447 L448 L450 L451 L452 L454 L455 L456 L458 L459 L460 L462 L463 L464 L466 L467 L468 L470 L471 L472 L474 L475 L476 L478 L479 L480 L482 L483 L484 L486 L487 L488 L490 L491 L492 L494 L495 L496 L498 L499 L500 L502 L503 L504 L506 L507 L508 L510 L511 L512 L514 L515 L516 L518 L519 L520 L522 L523 L524 L526 L527 L528 L530 L531 L532 L534 L535 L536 L538 L539 L540 L542 L543 L544 L546 L547 L548 L550 L551 L552 L554 L555 L556 L558 L559 L560 L562 L563 L564 L566 L567 L568 L570 L571 L572 L574 L575 L576 L578 L579 L580 L582 L583 L584 L586 L587 L588 L590 L591 L592 L594 L595 L596 L598 L599 L600 L602 L603 | A2 L612 L614 L615 | A2 A4 L612 L614 | A2 L0 L1 L3 L604 L606 L607 L608 L610 L611 L612 L614 L615 L616 L618 L619 L620 L622 L623 L624 L626 L627 L628 L630 L631 L632 L634 L635 L636 L638 L639 L640 L642 L643 L644 L646 L647 | A2 L616 L618 L619 | A2 A4 L616 L618 | A4 L612 L613 L614 | A2 A4 L608 L610 | A2 L608 L610 L611 | A4 L616 L617 L618 | A4 L608 L609 L610 | A2 L620 L622 L623 | A2 A4 L620 L622 | A2 A4 L604 L606 | A2 L604 L606 L607 | A4 L620 L621 L622 | A4 L604 L605 L606 | A2 L624 L626 L627 | A2 A4 L624 L626 | A2 A4 L1 L3 | A2 L0 L1 L3 | A4 L624 L625 L626 | A4 L1 L2 L3 | A2 L628 L630 L631 | A2 A4 L628 L630 | A2 A4 L644 L646 | A2 L644 L646 L647 | A4 L628 L629 L630 | A4 L644 L645 L646 | A2 L632 L634 L635 | A2 A4 L632 L634 | A2 A4 L640 L642 | A2 L640 L642 L643 | A4 L632 L633 L634 | A4 L640 L641 L642 | A2 L636 L638 L639 | A2 A4 L636 L638 | A4 L636 L637 L638 | A3 makes body 1 at (3980.1231, 2000, 398.2714) makes body 2 at (3930.3716, 2000, 393.293) in component "Inner Rotor Generator"
ref_plane "WorkPlane1" through (0, 0, 0) normal (0, -1, 0) x (-1, 0, 0)
sketch "Sketch1 (2)" plane through (0, 0, 0) normal (0, -1, 0) x (1, 0, 0)
  circle A0 centre (0, 0) radius 3600
  constraint coincident A0.centre origin
extrude "Extrude2" cut sketch "Sketch1 (2)" against normal blind 500 bodies 2 in component "Inner Rotor Generator"
ref_plane "WorkPlane2" through (0, 3000, 0) normal (0, 1, 0) x (1, 0, 0)
sketch "Sketch2" plane through (0, 3000, 0) normal (0, 1, 0) x (1, 0, 0)
  circle A0 centre (0, 0) radius 3600
  constraint coincident A0.centre origin
extrude "Extrude3" cut sketch "Sketch2" against normal blind 500 bodies 2 in component "Inner Rotor Generator"
sketch "Sketch1 (3)" plane through (0, 0, 0) normal (0, 1, 0) x (1, 0, 0) in component "Hub"
  circle A0 centre (0, 0) radius 1500
  constraint coincident A0.centre origin
extrude "Extrude1'" add sketch "Sketch1 (3)" against normal blind 4000 separate body makes body 3 in component "Hub"
ref_plane "WorkPlane1" through (0, -2176.1731, 1500) normal (0, 0, 1) x (1, 0, 0) in component "Hub"
sketch "Sketch2 (2)" plane through (0, -2176.1731, 1500) normal (0, 0, 1) x (1, 0, 0) in component "Hub"
  circle A0 centre (0, 300) radius 1000
extrude "Extrude2'" add sketch "Sketch2 (2)" along normal blind 700 and the other way blind 400 bodies 3 in component "Hub"
sketch "Sketch3" plane through (0, 0, 2200) normal (0, 0, 1) x (-1, 0, 0) in component "Hub"
  circle A0 centre (0, 1876.1731) radius 1000
  circle A1 centre (0, 1876.1731) radius 1500
  constraint concentric A0 A1
extrude "Extrude3'" add sketch "Sketch3" along normal blind 600 contours A0 | A1 bodies 3 in component "Hub"
sketch "Sketch4" plane through (0, 0, 2800) normal (0, 0, 1) x (-1, 0, 0) in component "Hub"
  circle A0 centre (0, 1876.1731) radius 1500
  circle A1 centre (0, 1876.1731) radius 875
  constraint concentric A0 A1
extrude "Extrude4" cut sketch "Sketch4" against normal blind 1400 contours A1 bodies 3 in component "Hub"
pattern_circular "C-Pattern1" count 3 over 360 about axis through (0, 1.75, 0) along (0, 1, 0) of "Extrude2'", "Extrude3'", "Extrude4" in component "Hub"
sketch "Sketch3 (2)" plane through (0, 500, 0) normal (0, -1, 0) x (1, 0, 0)
  line L0 (100, 994.9874) -> (100, 3598.6108)
  arc A0 (100, 3598.6108) -> (-100, 3598.6108) centre (0, 0) ccw
  line L1 (-100, 3598.6108) -> (-100, 994.9874)
  arc A1 (-100, 994.9874) -> (-410.8912, 911.6844) centre (0, 0) ccw
  line L2 (-410.8912, 911.6844) -> (-1712.7029, 3166.4884)
  arc A2 (-1712.7029, 3166.4884) -> (-1885.908, 3066.4884) centre (0, 0) ccw
  line L3 (-1885.908, 3066.4884) -> (-584.0963, 811.6844)
  arc A3 (-584.0963, 811.6844) -> (-811.6844, 584.0963) centre (0, 0) ccw
  line L4 (-811.6844, 584.0963) -> (-3066.4884, 1885.908)
  arc A4 (-3066.4884, 1885.908) -> (-3166.4884, 1712.7029) centre (0, 0) ccw
  line L5 (-3166.4884, 1712.7029) -> (-911.6844, 410.8912)
  arc A5 (-911.6844, 410.8912) -> (-994.9874, 100) centre (0, 0) ccw
  line L6 (-994.9874, 100) -> (-3598.6108, 100)
  arc A6 (-3598.6108, 100) -> (-3598.6108, -100) centre (0, 0) ccw
  line L7 (-3598.6108, -100) -> (-994.9874, -100)
  arc A7 (-994.9874, -100) -> (-911.6844, -410.8912) centre (0, 0) ccw
  line L8 (-911.6844, -410.8912) -> (-3166.4884, -1712.7029)
  arc A8 (-3166.4884, -1712.7029) -> (-3066.4884, -1885.908) centre (0, 0) ccw
  line L9 (-3066.4884, -1885.908) -> (-811.6844, -584.0963)
  arc A9 (-811.6844, -584.0963) -> (-584.0963, -811.6844) centre (0, 0) ccw
  line L10 (-584.0963, -811.6844) -> (-1885.908, -3066.4884)
  arc A10 (-1885.908, -3066.4884) -> (-1712.7029, -3166.4884) centre (0, 0) ccw
  line L11 (-1712.7029, -3166.4884) -> (-410.8912, -911.6844)
  arc A11 (-410.8912, -911.6844) -> (-100, -994.9874) centre (0, 0) ccw
  line L12 (-100, -994.9874) -> (-100, -3598.6108)
  arc A12 (-100, -3598.6108) -> (100, -3598.6108) centre (0, 0) ccw
  line L13 (100, -3598.6108) -> (100, -994.9874)
  arc A13 (100, -994.9874) -> (410.8912, -911.6844) centre (0, 0) ccw
  line L14 (410.8912, -911.6844) -> (1712.7029, -3166.4884)
  arc A14 (1712.7029, -3166.4884) -> (1885.908, -3066.4884) centre (0, 0) ccw
  line L15 (1885.908, -3066.4884) -> (584.0963, -811.6844)
  arc A15 (584.0963, -811.6844) -> (811.6844, -584.0963) centre (0, 0) ccw
  line L16 (811.6844, -584.0963) -> (3066.4884, -1885.908)
  arc A16 (3066.4884, -1885.908) -> (3166.4884, -1712.7029) centre (0, 0) ccw
  line L17 (3166.4884, -1712.7029) -> (911.6844, -410.8912)
  arc A17 (911.6844, -410.8912) -> (994.9874, -100) centre (0, 0) ccw
  line L18 (994.9874, -100) -> (3598.6108, -100)
  arc A18 (3598.6108, -100) -> (3598.6108, 100) centre (0, 0) ccw
  line L19 (3598.6108, 100) -> (994.9874, 100)
  arc A19 (994.9874, 100) -> (911.6844, 410.8912) centre (0, 0) ccw
  line L20 (911.6844, 410.8912) -> (3166.4884, 1712.7029)
  arc A20 (3166.4884, 1712.7029) -> (3066.4884, 1885.908) centre (0, 0) ccw
  line L21 (3066.4884, 1885.908) -> (811.6844, 584.0963)
  arc A21 (811.6844, 584.0963) -> (584.0963, 811.6844) centre (0, 0) ccw
  line L22 (584.0963, 811.6844) -> (1885.908, 3066.4884)
  arc A22 (1885.908, 3066.4884) -> (1712.7029, 3166.4884) centre (0, 0) ccw
  line L23 (1712.7029, 3166.4884) -> (410.8912, 911.6844)
  arc A23 (410.8912, 911.6844) -> (100, 994.9874) centre (0, 0) ccw
  circle A24 centre (0, 0) radius 500
  constraint concentric A18 A24
extrude "Extrude4'" cut sketch "Sketch3 (2)" against normal blind 2000 contours A24 bodies 2 in component "Inner Rotor Generator"
sketch "Sketch4 (2)" plane through (0, -4000, 0) normal (0, -1, 0) x (1, 0, 0)
  circle A0 centre (-9696.4454, -183.4467) radius 1500
  circle A1 centre (-9696.4454, -183.4467) radius 1000
  constraint concentric A0 A1
extrude "Extrude5" cut sketch "Sketch4 (2)" against normal blind 4100 contours A1 sketch seen with x (1, 0, 0) y (0, 1, 0) z (0, 0, 1) at (9696.4454, 0, 183.4467) bodies 3 in component "Hub"